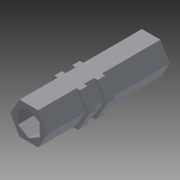
# Autodesk Inventor part: 3DR-Rod-Adapter-Enlightx-v2
Saved by Autodesk Inventor 2013 (Build 170138000, 138)
## iProperties
Created: 2013-08-23
Part Number: 3DR-Rod-Adapter-Enlightx-v2
Material: Generic
Document SubType Name: Modeling
Designer: Enlightx
Density: 1 g/cm^3
Author: Enlightx
Autodesk Inventor part; units mm, degrees
ref_plane "YZ Plane" through (0, 0, 0) normal (1, 0, 0) x (0, 1, 0)
ref_plane "XZ Plane" through (0, 0, 0) normal (0, 1, 0) x (-1, 0, 0)
ref_plane "XY Plane" through (0, 0, 0) normal (0, 0, 1) x (1, 0, 0)
sketch "Sketch2" plane through (0, 0, 0) normal (0, 1, 0) x (-1, 0, 0)
  line L0 (3.6373, 0) -> (1.8187, -3.15)
  line L1 (1.8187, -3.15) -> (-1.8187, -3.15)
  line L2 (-1.8187, -3.15) -> (-3.6373, 0)
  line L3 (-3.6373, 0) -> (-1.8187, 3.15)
  line L4 (-1.8187, 3.15) -> (1.8187, 3.15)
  line L5 (1.8187, 3.15) -> (3.6373, 0)
  point P0 (0, 0)
  point P1 (0, 0)
  dimension "d0" = 6.3
  constraints: 12 end point, 1 coincident, 13 other
  measures "d0" distance between parallel lines of L1 L4
extrude "Joint End" add sketch "Sketch2" along normal blind 7.5
sketch "Sketch3" plane through (0, 7.5, 0) normal (0, 1, 0) x (1, 0, 0)
  line L0 (4.3301, 0) -> (2.1651, -3.75)
  line L1 (2.1651, -3.75) -> (-2.1651, -3.75)
  line L2 (-2.1651, -3.75) -> (-4.3301, 0)
  line L3 (-4.3301, 0) -> (-2.1651, 3.75)
  line L4 (-2.1651, 3.75) -> (2.1651, 3.75)
  line L5 (2.1651, 3.75) -> (4.3301, 0)
  point P0 (0, 0)
  point P1 (0, 0)
  dimension "d3" = 7.5
  constraints: 12 end point, 1 coincident, 13 other
  measures "d3" distance between parallel lines of L1 L4
extrude "Spring Stop 1" add sketch "Sketch3" along normal blind 1.5
sketch "Sketch4" plane through (0, 9, 0) normal (0, 1, 0) x (1, 0, 0)
  line L0 (3.6373, 0) -> (1.8187, -3.15)
  line L1 (1.8187, -3.15) -> (-1.8187, -3.15)
  line L2 (-1.8187, -3.15) -> (-3.6373, 0)
  line L3 (-3.6373, 0) -> (-1.8187, 3.15)
  line L4 (-1.8187, 3.15) -> (1.8187, 3.15)
  line L5 (1.8187, 3.15) -> (3.6373, 0)
  point P0 (0, 0)
  point P1 (0, 0)
  point P2 (0, 0)
  dimension "d6" = 6.3
  constraints: 12 end point, 2 coincident, 13 other
  measures "d6" distance between parallel lines of L1 L4
extrude "Spring Slot" add sketch "Sketch4" along normal blind 2
sketch "Sketch5" plane through (0, 11, 0) normal (0, 1, 0) x (1, 0, 0)
  line L0 (4.3301, 0) -> (2.1651, -3.75)
  line L1 (2.1651, -3.75) -> (-2.1651, -3.75)
  line L2 (-2.1651, -3.75) -> (-4.3301, 0)
  line L3 (-4.3301, 0) -> (-2.1651, 3.75)
  line L4 (-2.1651, 3.75) -> (2.1651, 3.75)
  line L5 (2.1651, 3.75) -> (4.3301, 0)
  point P0 (0, 0)
  point P1 (0, 0)
  dimension "d9" = 7.5
  constraints: 12 end point, 1 coincident, 13 other
  measures "d9" distance between parallel lines of L1 L4
extrude "Spring Stop 2" add sketch "Sketch5" along normal blind 1.5
sketch "Sketch6" plane through (0, 12.5, 0) normal (0, 1, 0) x (1, 0, 0)
  line L0 (3.6373, 0) -> (1.8187, -3.15)
  line L1 (1.8187, -3.15) -> (-1.8187, -3.15)
  line L2 (-1.8187, -3.15) -> (-3.6373, 0)
  line L3 (-3.6373, 0) -> (-1.8187, 3.15)
  line L4 (-1.8187, 3.15) -> (1.8187, 3.15)
  line L5 (1.8187, 3.15) -> (3.6373, 0)
  point P0 (0, 0)
  point P1 (0, 0)
  dimension "d12" = 6.3
  constraints: 12 end point, 1 coincident, 13 other
  measures "d12" distance between parallel lines of L1 L4
extrude "Carbon End" add sketch "Sketch6" along normal blind 11.5
sketch "Sketch10" plane through (0, 0, 0) normal (0, -1, 0) x (1, 0, 0)
  line L0 (0, -2.4826) -> (-2.15, -1.2413)
  line L1 (-2.15, -1.2413) -> (-2.15, 1.2413)
  line L2 (-2.15, 1.2413) -> (0, 2.4826)
  line L3 (0, 2.4826) -> (2.15, 1.2413)
  line L4 (2.15, 1.2413) -> (2.15, -1.2413)
  line L5 (2.15, -1.2413) -> (0, -2.4826)
  point P0 (0, 0)
  point P1 (0, 0)
  dimension "d27" = 4.3
  constraints: 12 end point, 1 coincident, 13 other
  measures "d27" distance between parallel lines of L0 L3
extrude "Arm Hole" cut sketch "Sketch10" against normal blind 10
sketch "Sketch11" plane through (0, 24, 0) normal (0, 1, 0) x (1, 0, 0)
  line L0 (0, -1.8475) -> (-1.6, -0.9238)
  line L1 (-1.6, -0.9238) -> (-1.6, 0.9238)
  line L2 (-1.6, 0.9238) -> (0, 1.8475)
  line L3 (0, 1.8475) -> (1.6, 0.9238)
  line L4 (1.6, 0.9238) -> (1.6, -0.9238)
  line L5 (1.6, -0.9238) -> (0, -1.8475)
  point P0 (0, 0)
  point P1 (0, 0)
  dimension "d30" = 3.2
  dimension "d31" = 3.695
  constraints: 12 end point, 1 coincident, 13 other
  measures "d30" distance between parallel lines of L5 L2
  measures "d31" distance of L0.start L2.end
extrude "Carbon Hole" cut sketch "Sketch11" against normal blind 10
sketch "Sketch12" plane through (0, 12.5, 0) normal (0, 1, 0) x (1, 0, 0)
  line L0 (2.1651, -3.75) -> (4.3301, 0) projected
  line L1 (-4.3301, 0) -> (-2.1651, -3.75) projected
  line L2 (-2.1651, -3.75) -> (2.1651, -3.75) projected
  line L3 (-2.5115, -3.15) -> (2.5115, -3.15)
  line L4 (2.5115, -3.15) -> (2.1651, -3.75)
  line L5 (2.1651, -3.75) -> (-2.1651, -3.75)
  line L6 (-2.1651, -3.75) -> (-2.5115, -3.15)
  point P0 (0, 0)
  constraints: 8 end point, 3 collinear, 2 point on line, 1 parallel
extrude "Bottom Cutout" cut sketch "Sketch12" against normal blind 5
body "Solid1"
